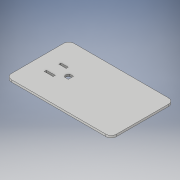
# Autodesk Inventor part: top
Saved by Autodesk Inventor 2019 (Build 230136000, 136)
## iProperties
Created: 2022-02-05
Part Number: top
Material: Generic
Document SubType Name: Modeling
Designer: josec
Density: 1 g/cm^3
Appearance: Default
Author: josec
Autodesk Inventor part; units mm, degrees
ref_plane "YZ Plane" through (0, 0, 0) normal (1, 0, 0) x (0, 1, 0)
ref_plane "XZ Plane" through (0, 0, 0) normal (0, 1, 0) x (-1, 0, 0)
ref_plane "XY Plane" through (0, 0, 0) normal (0, 0, 1) x (1, 0, 0)
sketch "Sketch1" plane through (0, 0, 0) normal (0, 1, 0) x (-1, 0, 0)
  line L0 (5, 0) -> (95.5, 0)
  line L1 (100.5, -5) -> (100.5, -55)
  line L2 (95.5, -60) -> (5, -60)
  line L3 (0, -55) -> (0, -5)
  arc A0 (100.5, -2) -> (98.5, 0) centre (98.5, -2) ccw
  arc A1 (5, 0) -> (0, -5) centre (5, -5) ccw
  arc A2 (95.5, -60) -> (100.5, -55) centre (95.5, -55) ccw
  arc A3 (0, -55) -> (5, -60) centre (5, -55) ccw
  arc A4 (100.5, -5) -> (95.5, 0) centre (95.5, -5) ccw
  point P0 (0, 0)
  point P1 (100.5, -60)
  point P2 (100.5, 0)
  point P3 (0, -60)
  dimension "d0" = 100.5
  dimension "d1" = 60
  dimension "d2" = 2
  dimension "d3" = 5
  constraints: 10 point on circle, 10 point on line, 10 tangent, 8 end point, 5 centre point, 3 equal radius, 2 parallel, 1 horizontal, 1 perpendicular
  measures "d0" distance of point (100.5, -60) point (0, -60)
  measures "d1" distance of point (100.5, 0) point (100.5, -60)
  measures "d2" radius of A0
  measures "d3" radius of A1
extrude "Extrusion1" add sketch "Sketch1" along normal blind 2
sketch "Sketch2" plane through (0, 2, 0) normal (0, 1, 0) x (1, 0, 0)
  line L0 (0, 0) -> (-100.5, 0) construction
  line L1 (-100.5, 0) -> (-100.5, 60) construction
  line L2 (-100.5, 60) -> (0, 60) construction
  line L3 (0, 60) -> (0, 0) construction
  line L4 (-100.5, 55) -> (-100.5, 5) construction
  line L5 (-100.5, 30) -> (-97.5, 30) construction
  line L6 (-97.5, 30) -> (-97.5, 41.5) construction
  line L7 (-97.5, 41.5) -> (-60.5, 41.5) construction
  line L8 (-60.5, 41.5) -> (-60.5, 18.5) construction
  line L9 (-60.5, 18.5) -> (-97.5, 18.5) construction
  line L10 (-97.5, 18.5) -> (-97.5, 41.5) construction
  line L11 (-97.5, 18.5) -> (-86.5, 18.5) construction
  line L12 (-86.5, 18.5) -> (-86.5, 22.5) construction
  line L13 (-86.5, 22.5) -> (-97.5, 22.5) construction
  line L14 (-97.5, 22.5) -> (-97.5, 18.5) construction
  line L15 (-86.5, 22.5) -> (-78, 22.5)
  line L16 (-78, 22.5) -> (-78, 24.5)
  line L17 (-78, 24.5) -> (-86.5, 24.5)
  line L18 (-86.5, 24.5) -> (-86.5, 22.5)
  line L19 (-97.5, 41.5) -> (-97.5, 37.5) construction
  line L20 (-97.5, 37.5) -> (-85.5, 37.5) construction
  line L21 (-85.5, 37.5) -> (-78.5, 37.5)
  line L22 (-78.5, 37.5) -> (-78.5, 35.5)
  line L23 (-78.5, 35.5) -> (-85.5, 35.5)
  line L24 (-85.5, 35.5) -> (-85.5, 37.5)
  line L25 (-60.5, 30) -> (-68.5, 30) construction
  line L26 (-68.5, 30) -> (-68.5, 32.5) construction
  line L27 (-68.5, 32.5) -> (-72, 32.5)
  line L28 (-68.5, 27.5) -> (-68.5, 32.5)
  line L29 (-68.5, 32.5) -> (-72, 32.5) construction
  line L30 (-72, 32.5) -> (-72, 27.5) construction
  arc A0 (-72, 32.5) -> (-72, 27.5) centre (-70.6667, 30) ccw
  line L31 (-72, 27.5) -> (-68.5, 27.5)
  dimension "d6" = 100.5
  dimension "d7" = 60
  dimension "d8" = 3
  dimension "d9" = 11.5
  dimension "d10" = 37
  dimension "d11" = 23
  dimension "d12" = 11
  dimension "d13" = 4
  dimension "d14" = 8.5
  dimension "d15" = 2
  dimension "d16" = 4
  dimension "d17" = 12
  dimension "d18" = 7
  dimension "d19" = 2
  dimension "d20" = 8
  dimension "d21" = 2.5
  dimension "d24" = 3.5
  constraints: 62 end point, 10 parallel, 9 horizontal, 6 perpendicular, 2 midpoint, 2 point on circle, 2 vertical, 1 centre point, 1 point on line
  measures "d6" distance of L1.end L2.end
  measures "d7" distance of L0.end L1.end
  measures "d8" distance of L5.start L5.end
  measures "d9" distance of L5.end L6.end
  measures "d10" distance of L8.end L9.end
  measures "d11" distance of L7.end L8.end
  measures "d12" distance of L13.end L12.end
  measures "d13" distance of L12.end L11.end
  measures "d14" distance of L17.end L16.end
  measures "d15" distance of L16.end L15.end
  measures "d16" distance of L6.end L19.end
  measures "d17" distance of L19.end L20.end
  measures "d18" distance of L22.end L23.end
  measures "d19" distance of L21.end L22.end
  measures "d20" distance of L25.start L25.end
  measures "d21" distance of L25.end L26.end
  measures "d24" distance of L27.end L26.end
extrude "Extrusion2" cut sketch "Sketch2" against normal blind 2
body "Solid1"
